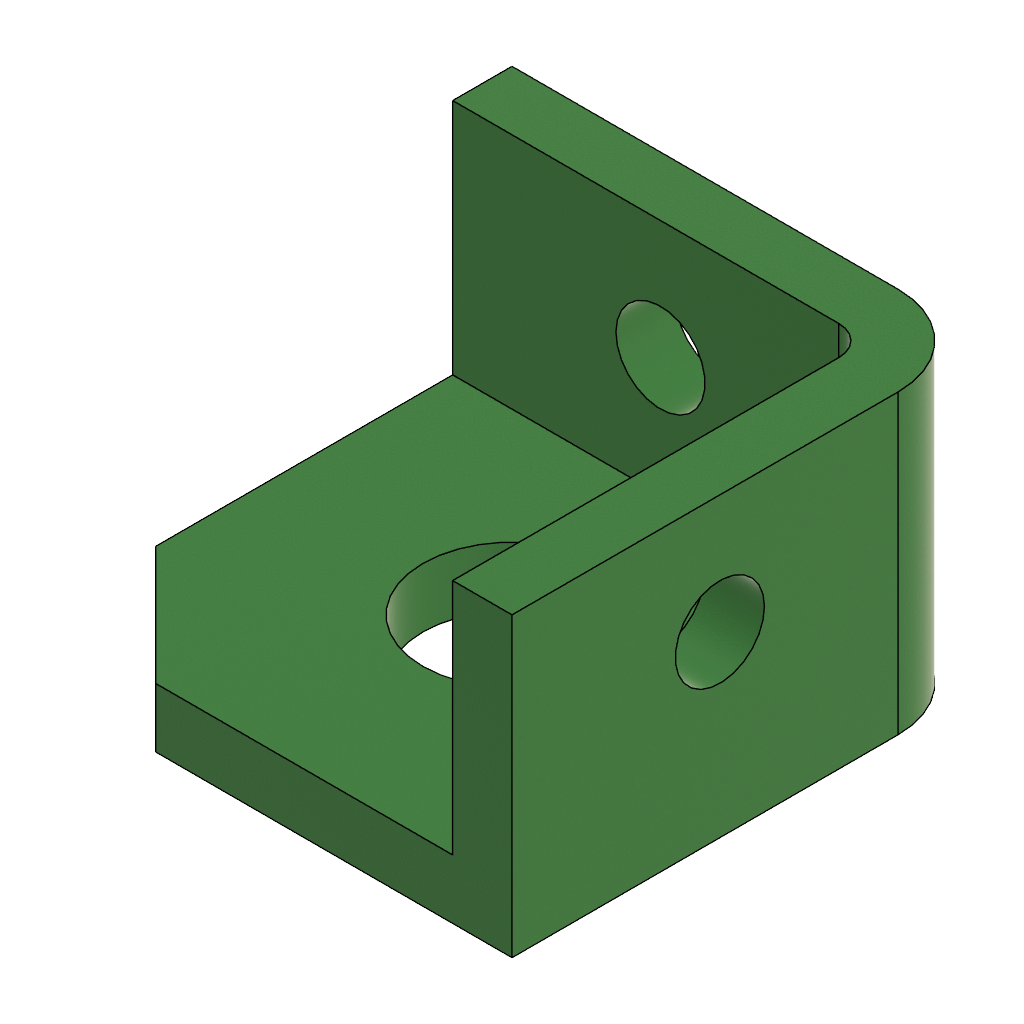
Bracket (Autodesk Fusion 360 design; units mm, degrees)
part number: 2026-01-26-22-07-11-482
Autodesk Fusion 360 part; units mm, degrees
sketch "Sketch1" plane through (0, 0, 0) normal (0, 0, 1) x (1, 0, 0)
  line L0 (0, 0) -> (80, 0)
  line L1 (80, 0) -> (80, 80)
  line L2 (80, 80) -> (0, 80)
  line L3 (0, 80) -> (0, 0)
  line L4 (0, 20) -> (20, 0)
  circle A0 centre (40, 40) radius 15
  dimension "d1" = 80
  dimension "d2" = 80
  dimension "d3" = 20
  dimension "d4" = 20
  dimension "d5" = 30
  dimension "d6" = 40
  dimension "d7" = 40
  constraint horizontal L0
  constraint vertical L1
  constraint horizontal L2
  constraint vertical L3
  constraint coincident L0.start L3.end
  constraint coincident L3 L4.start
  constraint coincident L0 L4.end
  measures "d1" distance of L0.start L0.end
  measures "d2" distance of L0.start L2.end
  measures "d3" distance of L0.start L4.start
  measures "d4" distance of L0.start L4.end
  measures "d5" diameter of A0
  measures "d6" distance of L3 A0.centre
  measures "d7" distance of L0 A0.centre
extrude "Extrude1" add sketch "Sketch1" along normal blind 10 contours L0 L1 L2 L3 L4
sketch "Sketch2" plane through (0, 0, 10) normal (0, 0, 1) x (-1, 0, 0)
  circle A0 centre (-40, -40) radius 15
  line L0 (0, -20) -> (-20, 0)
  line L1 (-20, 0) -> (-80, 0)
  line L2 (-80, 0) -> (-80, -80)
  line L3 (-80, -80) -> (0, -80)
  line L4 (0, -80) -> (0, -20)
  line L5 (0, -80) -> (-80, -80)
  line L6 (-80, -80) -> (-80, -70)
  line L7 (-80, -70) -> (0, -70)
  line L8 (0, -70) -> (0, -80)
  line L9 (-80, -80) -> (-70, -80)
  line L10 (-70, -80) -> (-70, 0)
  line L11 (-70, 0) -> (-80, 0)
  line L12 (-80, 0) -> (-80, -80)
  dimension "d10" = 10
  dimension "d11" = 10
  constraint horizontal L5
  constraint vertical L6
  constraint horizontal L7
  constraint vertical L8
  constraint coincident L2 L6.end
  constraint coincident L3.end L4.start
  constraint horizontal L9
  constraint vertical L10
  constraint horizontal L11
  constraint vertical L12
  constraint coincident L1 L10.end
  measures "d10" distance of L3.end L7.end
  measures "d11" distance of L10.end L1.end
extrude "Extrude2" add sketch "Sketch2" along normal blind 40 contours L3 L4 L5 L7 L8 L10 | L1 L2 L7 L10 L11 L12 | L2 L3 L5 L6 L7 L9 L10 L12
fillet "Fillet1" radius 5 1 edges at (70, 70, 30)
fillet "Fillet2" radius 15 1 edges at (80, 80, 25)
hole "Hole1" at (70, 32.5, 30) direction (1, 0, 0) diameter 15 depth 25 tip angle 118
delete_face "DeleteFace1" 1 faces at (73.3333, 32.8738, 37.4907)
hole "Hole2" at (70, 41.1757, 28.9917) direction (1, 0, 0) diameter 15 depth 25 tip angle 118
sketch "Sketch3" plane through (0, 0, 0) normal (0, 0, 1) x (1, 0, 0)
delete_face "DeleteFace2" 1 faces at (73.3333, 41.5496, 36.4824)
sketch "Sketch4" plane through (70, 0, 0) normal (-1, 0, 0) x (0, -1, 0)
  line L0 (-65, 50) -> (-65, 10)
  line L1 (-65, 10) -> (0, 10)
  line L2 (0, 10) -> (0, 50)
  line L3 (0, 50) -> (-65, 50)
  circle A0 centre (-35, 30) radius 7.5
  dimension "d24" = 15
  dimension "d25" = 35
  dimension "d26" = 20
  measures "d24" diameter of A0
  measures "d25" distance of L2 A0.centre
  measures "d26" distance of L1 A0.centre
extrude "Extrude3" cut sketch "Sketch4" against normal blind 10 contours A0
sketch "Sketch5" plane through (0, 70, 0) normal (0, -1, 0) x (1, 0, 0)
  line L0 (65, 10) -> (65, 50)
  line L1 (65, 50) -> (0, 50)
  line L2 (0, 50) -> (0, 10)
  line L3 (0, 10) -> (65, 10)
  circle A0 centre (35, 30) radius 7.5
  dimension "d29" = 15
  dimension "d31" = 20
  dimension "d32" = 35
  measures "d29" diameter of A0
  measures "d31" distance of L3 A0.centre
  measures "d32" distance of L2 A0.centre
extrude "Extrude4" cut sketch "Sketch5" against normal blind 10 contours A0
